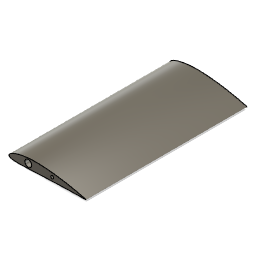
Airfoil v6 (Autodesk Fusion 360 design; units mm, degrees)
Autodesk Fusion 360 part; units mm, degrees
sketch "Esquisse7" plane through (0, 0, 0) normal (0, 0, 1) x (1, 0, 0)
  spline S0 degree 5 poles (0, 0) (-0.0102, 0.0513) (-0.0251, 0.1551) (-0.0316, 0.3133) (-0.0088, 0.5269) (0.0656, 0.7917) (0.1767, 1.0474) (0.3135, 1.2879) (0.4648, 1.5082) (0.6211, 1.7053) (0.7754, 1.8785) (0.9248, 2.03) (1.0699, 2.1643) (1.2127, 2.2866) (1.3565, 2.4023) (1.5042, 2.516) (1.6573, 2.63) (1.8156, 2.7448) (1.9781, 2.8596) (2.143, 2.9726) (2.3089, 3.0823) (2.4745, 3.1876) (2.6395, 3.2884) (2.8042, 3.3853) (2.969, 3.4791) (3.1347, 3.5708) (3.3016, 3.6612) (3.4698, 3.7505) (3.6393, 3.8389) (3.8097, 3.9259) (3.9807, 4.0114) (4.1521, 4.0951) (4.3237, 4.177) (4.4955, 4.2571) (4.6676, 4.3356) (4.8401, 4.4128) (5.0131, 4.4888) (5.1866, 4.5637) (5.3605, 4.6375) (5.535, 4.7103) (5.7098, 4.7821) (5.8849, 4.8527) (6.0602, 4.9221) (6.2358, 4.9905) (6.4117, 5.0579) (6.5879, 5.1242) (6.7643, 5.1896) (6.941, 5.2541) (7.118, 5.3178) (7.2952, 5.3805) (7.4727, 5.4424) (7.6504, 5.5035) (7.8284, 5.5637) (8.0065, 5.6231) (8.1849, 5.6816) (8.3634, 5.7394) (8.5421, 5.7964) (8.7211, 5.8527) (8.9002, 5.9082) (9.0795, 5.963) (9.259, 6.0171) (9.4387, 6.0704) (9.6185, 6.1231) (9.7985, 6.1751) (9.9786, 6.2264) (10.1589, 6.277) (10.3393, 6.3269) (10.5199, 6.3763) (10.7006, 6.4249) (10.8815, 6.473) (11.0625, 6.5204) (11.2436, 6.5672) (11.4249, 6.6134) (11.6063, 6.659) (11.7878, 6.704) (11.9694, 6.7484) (12.1512, 6.7923) (12.333, 6.8355) (12.515, 6.8782) (12.6971, 6.9204) (12.8793, 6.9619) (13.0616, 7.003) (13.2439, 7.0434) (13.4264, 7.0834) (13.609, 7.1228) (13.7917, 7.1617) (13.9745, 7.2) (14.1574, 7.2378) (14.3403, 7.2752) (14.5233, 7.312) (14.7065, 7.3482) (14.8897, 7.384) (15.073, 7.4193) (15.2563, 7.4541) (15.4398, 7.4884) (15.6233, 7.5223) (15.8069, 7.5556) (15.9906, 7.5885) (16.1743, 7.6209) (16.3581, 7.6528) (16.542, 7.6842) (16.726, 7.7152) (16.91, 7.7457) (17.0941, 7.7758) (17.2782, 7.8054) (17.4624, 7.8345) (17.6466, 7.8632) (17.831, 7.8915) (18.0153, 7.9193) (18.1998, 7.9467) (18.3842, 7.9736) (18.5688, 8.0001) (18.7534, 8.0262) (18.938, 8.0519) (19.1227, 8.0771) (19.3074, 8.1019) (19.4922, 8.1262) (19.677, 8.1502) (19.8619, 8.1737) (20.0468, 8.1968) (20.2318, 8.2195) (20.4168, 8.2418) (20.6018, 8.2637) (20.7869, 8.2852) (20.972, 8.3062) (21.1572, 8.3269) (21.3424, 8.3472) (21.5276, 8.3671) (21.7129, 8.3866) (21.8982, 8.4056) (22.0835, 8.4243) (22.2689, 8.4426) (22.4543, 8.4606) (22.6397, 8.4781) (22.8251, 8.4952) (23.0106, 8.512) (23.1961, 8.5284) (23.3817, 8.5444) (23.5673, 8.56) (23.7528, 8.5753) (23.9385, 8.5902) (24.1241, 8.6047) (24.3098, 8.6188) (24.4954, 8.6326) (24.6812, 8.646) (24.8669, 8.659) (25.0526, 8.6717) (25.2384, 8.684) (25.4242, 8.696) (25.61, 8.7076) (25.7958, 8.7188) (25.9816, 8.7297) (26.1675, 8.7402) (26.3534, 8.7504) (26.5392, 8.7602) (26.7251, 8.7696) (26.9111, 8.7788) (27.097, 8.7875) (27.2829, 8.796) (27.4689, 8.804) (27.6548, 8.8118) (27.8408, 8.8191) (28.0268, 8.8262) (28.2127, 8.8329) (28.3987, 8.8393) (28.5847, 8.8453) (28.7707, 8.851) (28.9567, 8.8563) (29.1428, 8.8614) (29.3288, 8.8661) (29.5148, 8.8704) (29.7009, 8.8744) (29.8869, 8.8781) (30.0729, 8.8815) (30.259, 8.8845) (30.445, 8.8873) (30.6311, 8.8896) (30.8171, 8.8917) (31.0032, 8.8934) (31.1892, 8.8949) (31.3753, 8.896) (31.5613, 8.8967) (31.7473, 8.8972) (31.9334, 8.8973) (32.1194, 8.8972) (32.3055, 8.8967) (32.4915, 8.8959) (32.6775, 8.8947) (32.8636, 8.8933) (33.0496, 8.8916) (33.2356, 8.8895) (33.4216, 8.8871) (33.6076, 8.8844) (33.7936, 8.8815) (33.9795, 8.8782) (34.1655, 8.8745) (34.3515, 8.8706) (34.5375, 8.8664) (34.7235, 8.8619) (34.9095, 8.8571) (35.0955, 8.852) (35.2814, 8.8466) (35.4672, 8.8408) (35.6529, 8.8348) (35.8384, 8.8284) (36.0237, 8.8218) (36.2087, 8.8149) (36.3935, 8.8079) (36.5781, 8.8006) (36.7625, 8.7931) (36.9468, 8.7854) (37.131, 8.7775) (37.3152, 8.7695) (37.4995, 8.7612) (37.6838, 8.7528) (37.8681, 8.7442) (38.0525, 8.7353) (38.2369, 8.7263) (38.4212, 8.7171) (38.6055, 8.7078) (38.7898, 8.6982) (38.974, 8.6885) (39.1583, 8.6786) (39.3425, 8.6685) (39.5267, 8.6582) (39.711, 8.6477) (39.8952, 8.6371) (40.0794, 8.6262) (40.2637, 8.6152) (40.4479, 8.604) (40.632, 8.5927) (40.8162, 8.5811) (41.0004, 8.5694) (41.1845, 8.5575) (41.3687, 8.5455) (41.5528, 8.5332) (41.7369, 8.5208) (41.921, 8.5082) (42.1051, 8.4955) (42.2892, 8.4825) (42.4733, 8.4694) (42.6574, 8.4561) (42.8414, 8.4427) (43.0255, 8.4291) (43.2095, 8.4153) (43.3935, 8.4013) (43.5775, 8.3872) (43.7615, 8.3729) (43.9455, 8.3585) (44.1295, 8.3439) (44.3135, 8.3291) (44.4974, 8.3141) (44.6813, 8.299) (44.8653, 8.2837) (45.0492, 8.2683) (45.2331, 8.2527) (45.4169, 8.2369) (45.6008, 8.221) (45.7847, 8.2049) (45.9685, 8.1886) (46.1523, 8.1722) (46.3362, 8.1556) (46.52, 8.1389) (46.7037, 8.122) (46.8875, 8.1049) (47.0713, 8.0877) (47.255, 8.0704) (47.4388, 8.0528) (47.6225, 8.0352) (47.8062, 8.0173) (47.9899, 7.9993) (48.1735, 7.9812) (48.3572, 7.9629) (48.5408, 7.9444) (48.7245, 7.9258) (48.9081, 7.907) (49.0917, 7.8881) (49.2753, 7.869) (49.4589, 7.8498) (49.6424, 7.8304) (49.826, 7.8109) (50.0095, 7.7912) (50.193, 7.7713) (50.3765, 7.7514) (50.56, 7.7312) (50.7434, 7.7109) (50.9269, 7.6905) (51.1103, 7.6699) (51.2937, 7.6492) (51.4771, 7.6283) (51.6605, 7.6073) (51.8439, 7.5861) (52.0272, 7.5648) (52.2106, 7.5433) (52.3939, 7.5217) (52.5772, 7.4999) (52.7605, 7.478) (52.9438, 7.4559) (53.127, 7.4337) (53.3102, 7.4114) (53.4935, 7.3889) (53.6767, 7.3663) (53.8599, 7.3435) (54.043, 7.3206) (54.2262, 7.2975) (54.4093, 7.2743) (54.5924, 7.2509) (54.7755, 7.2274) (54.9586, 7.2038) (55.1417, 7.18) (55.3247, 7.1561) (55.5078, 7.132) (55.6908, 7.1078) (55.8738, 7.0835) (56.0567, 7.059) (56.2397, 7.0344) (56.4226, 7.0096) (56.6056, 6.9847) (56.7885, 6.9597) (56.9714, 6.9345) (57.1542, 6.9091) (57.3371, 6.8837) (57.5199, 6.8581) (57.7027, 6.8323) (57.8855, 6.8065) (58.0683, 6.7805) (58.2511, 6.7543) (58.4338, 6.728) (58.6165, 6.7016) (58.7992, 6.675) (58.9819, 6.6483) (59.1646, 6.6215) (59.3472, 6.5945) (59.5298, 6.5674) (59.7125, 6.5402) (59.895, 6.5128) (60.0776, 6.4853) (60.2602, 6.4576) (60.4427, 6.4298) (60.6252, 6.4019) (60.8077, 6.3739) (60.9902, 6.3457) (61.1726, 6.3174) (61.3551, 6.2889) (61.5375, 6.2603) (61.7199, 6.2316) (61.9022, 6.2027) (62.0846, 6.1737) (62.2669, 6.1446) (62.4492, 6.1153) (62.6315, 6.086) (62.8138, 6.0564) (62.996, 6.0268) (63.1783, 5.997) (63.3605, 5.9671) (63.5427, 5.937) (63.7248, 5.9068) (63.907, 5.8765) (64.0891, 5.846) (64.2712, 5.8155) (64.4533, 5.7848) (64.6354, 5.7539) (64.8174, 5.7229) (64.9995, 5.6918) (65.1815, 5.6606) (65.3634, 5.6292) (65.5454, 5.5977) (65.7273, 5.5661) (65.9092, 5.5343) (66.0911, 5.5024) (66.273, 5.4704) (66.4549, 5.4382) (66.6367, 5.406) (66.8185, 5.3736) (67.0003, 5.341) (67.1821, 5.3083) (67.3638, 5.2755) (67.5455, 5.2426) (67.7272, 5.2095) (67.9089, 5.1763) (68.0906, 5.143) (68.2722, 5.1096) (68.4538, 5.076) (68.6354, 5.0423) (68.8169, 5.0084) (68.9985, 4.9744) (69.18, 4.9403) (69.3615, 4.9061) (69.543, 4.8718) (69.7244, 4.8373) (69.9059, 4.8027) (70.0873, 4.7679) (70.2686, 4.733) (70.45, 4.698) (70.6313, 4.6629) (70.8127, 4.6276) (70.9939, 4.5922) (71.1752, 4.5567) (71.3564, 4.5211) (71.5377, 4.4853) (71.7189, 4.4494) (71.9, 4.4133) (72.0812, 4.3772) (72.2623, 4.3409) (72.4434, 4.3045) (72.6245, 4.2679) (72.8055, 4.2312) (72.9865, 4.1944) (73.1675, 4.1575) (73.3485, 4.1204) (73.5295, 4.0832) (73.7104, 4.0459) (73.8913, 4.0084) (74.0722, 3.9708) (74.253, 3.9331) (74.4339, 3.8953) (74.6147, 3.8573) (74.7954, 3.8192) (74.9762, 3.781) (75.1569, 3.7426) (75.3376, 3.7041) (75.5183, 3.6655) (75.6989, 3.6268) (75.8796, 3.5879) (76.0602, 3.5489) (76.2407, 3.5098) (76.4213, 3.4705) (76.6018, 3.4311) (76.7823, 3.3916) (76.9628, 3.3519) (77.1432, 3.3122) (77.3236, 3.2722) (77.504, 3.2322) (77.6844, 3.192) (77.8647, 3.1517) (78.045, 3.1113) (78.2253, 3.0707) (78.4056, 3.03) (78.5858, 2.9892) (78.766, 2.9483) (78.9462, 2.9072) (79.1264, 2.866) (79.3065, 2.8246) (79.4866, 2.7831) (79.6666, 2.7415) (79.8467, 2.6998) (80.0267, 2.6579) (80.2067, 2.6159) (80.3866, 2.5738) (80.5666, 2.5316) (80.7465, 2.4892) (80.9263, 2.4466) (81.1062, 2.404) (81.2859, 2.3612) (81.4657, 2.3182) (81.6455, 2.2752) (81.8252, 2.232) (82.0049, 2.1887) (82.1847, 2.1453) (82.3643, 2.1017) (82.544, 2.058) (82.7235, 2.0142) (82.903, 1.9701) (83.0824, 1.926) (83.2618, 1.8817) (83.4412, 1.8373) (83.6208, 1.7928) (83.8003, 1.7483) (83.98, 1.7036) (84.1595, 1.6588) (84.3389, 1.6138) (84.518, 1.5685) (84.6968, 1.5229) (84.8754, 1.4772) (85.0541, 1.4313) (85.2332, 1.3855) (85.4128, 1.3399) (85.5929, 1.2945) (85.7733, 1.2492) (85.9534, 1.2035) (86.1326, 1.1573) (86.3106, 1.1101) (86.4872, 1.0621) (86.663, 1.0135) (86.8393, 0.9651) (87.0176, 0.9177) (87.1988, 0.8719) (87.3831, 0.8277) (87.569, 0.7843) (87.7535, 0.7401) (87.9336, 0.6931) (88.1067, 0.642) (88.2727, 0.5866) (88.4345, 0.5288) (88.5991, 0.4726) (88.7741, 0.4223) (88.9652, 0.3811) (89.1737, 0.3493) (89.3935, 0.3227) (89.61, 0.292) (89.8042, 0.2472) (89.9561, 0.181) (90.0488, 0.0924) (90.0719, -0.0084) (90.0246, -0.1002) (89.9133, -0.1623) (89.7503, -0.1873) (89.5518, -0.1807) (89.3352, -0.1543) (89.1161, -0.123) (88.9064, -0.0997) (88.7111, -0.0903) (88.529, -0.094) (88.3554, -0.1064) (88.1842, -0.1213) (88.0098, -0.133) (87.8296, -0.139) (87.6438, -0.1392) (87.4543, -0.1358) (87.2637, -0.1313) (87.0746, -0.1282) (86.8879, -0.1277) (86.7036, -0.1296) (86.521, -0.1331) (86.3389, -0.1371) (86.1561, -0.1406) (85.9723, -0.143) (85.7875, -0.1444) (85.602, -0.1451) (85.4164, -0.1457) (85.231, -0.1465) (85.0461, -0.1478) (84.8616, -0.1496) (84.6775, -0.1518) (84.4934, -0.154) (84.3093, -0.1562) (84.1249, -0.1581) (83.9404, -0.16) (83.7558, -0.1617) (83.5711, -0.1634) (83.3866, -0.1652) (83.2021, -0.1671) (83.0177, -0.1691) (82.8334, -0.1712) (82.6491, -0.1734) (82.4648, -0.1755) (82.2805, -0.1777) (82.0961, -0.1798) (81.9118, -0.1819) (81.7274, -0.1841) (81.5431, -0.1863) (81.3588, -0.1886) (81.1745, -0.1909) (80.9903, -0.1932) (80.8061, -0.1956) (80.6219, -0.198) (80.4377, -0.2004) (80.2535, -0.2029) (80.0693, -0.2054) (79.8851, -0.2079) (79.7009, -0.2104) (79.5168, -0.213) (79.3326, -0.2156) (79.1485, -0.2183) (78.9644, -0.221) (78.7803, -0.2237) (78.5962, -0.2264) (78.4122, -0.2292) (78.2281, -0.232) (78.0441, -0.2348) (77.86, -0.2377) (77.676, -0.2406) (77.492, -0.2436) (77.308, -0.2465) (77.124, -0.2495) (76.9401, -0.2526) (76.7561, -0.2556) (76.5722, -0.2588) (76.3882, -0.2619) (76.2043, -0.2651) (76.0204, -0.2683) (75.8365, -0.2715) (75.6526, -0.2748) (75.4688, -0.2781) (75.2849, -0.2814) (75.1011, -0.2848) (74.9173, -0.2882) (74.7334, -0.2917) (74.5496, -0.2951) (74.3658, -0.2987) (74.1821, -0.3022) (73.9983, -0.3058) (73.8145, -0.3094) (73.6308, -0.3131) (73.4471, -0.3167) (73.2633, -0.3205) (73.0796, -0.3242) (72.8959, -0.328) (72.7123, -0.3318) (72.5286, -0.3357) (72.3449, -0.3396) (72.1613, -0.3435) (71.9776, -0.3475) (71.794, -0.3515) (71.6104, -0.3555) (71.4268, -0.3596) (71.2432, -0.3637) (71.0596, -0.3678) (70.8761, -0.372) (70.6925, -0.3762) (70.509, -0.3804) (70.3254, -0.3847) (70.1419, -0.389) (69.9584, -0.3933) (69.7749, -0.3977) (69.5914, -0.4021) (69.408, -0.4066) (69.2245, -0.4111) (69.041, -0.4156) (68.8576, -0.4201) (68.6742, -0.4247) (68.4908, -0.4293) (68.3074, -0.434) (68.124, -0.4387) (67.9406, -0.4434) (67.7572, -0.4481) (67.5739, -0.4529) (67.3905, -0.4578) (67.2072, -0.4626) (67.0238, -0.4675) (66.8405, -0.4724) (66.6572, -0.4774) (66.4739, -0.4824) (66.2906, -0.4874) (66.1074, -0.4925) (65.9241, -0.4976) (65.7409, -0.5027) (65.5576, -0.5079) (65.3744, -0.5131) (65.1912, -0.5183) (65.008, -0.5236) (64.8248, -0.5289) (64.6416, -0.5342) (64.4584, -0.5396) (64.2753, -0.545) (64.0921, -0.5504) (63.909, -0.5558) (63.7258, -0.5613) (63.5427, -0.5669) (63.3596, -0.5724) (63.1765, -0.578) (62.9934, -0.5836) (62.8103, -0.5893) (62.6273, -0.595) (62.4442, -0.6007) (62.2612, -0.6064) (62.0781, -0.6122) (61.8951, -0.618) (61.7121, -0.6239) (61.5291, -0.6297) (61.3461, -0.6356) (61.1631, -0.6416) (60.9801, -0.6475) (60.7971, -0.6535) (60.6142, -0.6596) (60.4312, -0.6656) (60.2483, -0.6717) (60.0654, -0.6778) (59.8825, -0.6839) (59.6996, -0.6901) (59.5167, -0.6963) (59.3338, -0.7025) (59.1509, -0.7088) (58.968, -0.7151) (58.7852, -0.7214) (58.6023, -0.7277) (58.4195, -0.7341) (58.2367, -0.7405) (58.0539, -0.7469) (57.8711, -0.7534) (57.6883, -0.7599) (57.5055, -0.7664) (57.3227, -0.7729) (57.1399, -0.7795) (56.9572, -0.786) (56.7744, -0.7927) (56.5917, -0.7993) (56.4089, -0.8059) (56.2262, -0.8126) (56.0435, -0.8193) (55.8608, -0.8261) (55.6781, -0.8328) (55.4954, -0.8396) (55.3127, -0.8464) (55.1301, -0.8532) (54.9474, -0.8601) (54.7648, -0.867) (54.5821, -0.8739) (54.3995, -0.8808) (54.2169, -0.8877) (54.0343, -0.8947) (53.8517, -0.9017) (53.6691, -0.9087) (53.4865, -0.9157) (53.3039, -0.9228) (53.1213, -0.9298) (52.9388, -0.9369) (52.7562, -0.944) (52.5737, -0.9511) (52.3911, -0.9583) (52.2086, -0.9654) (52.0261, -0.9726) (51.8436, -0.9798) (51.6611, -0.987) (51.4786, -0.9943) (51.2961, -1.0015) (51.1136, -1.0088) (50.9311, -1.0161) (50.7487, -1.0233) (50.5662, -1.0307) (50.3838, -1.038) (50.2013, -1.0453) (50.0189, -1.0527) (49.8365, -1.0601) (49.6541, -1.0674) (49.4717, -1.0748) (49.2893, -1.0822) (49.1069, -1.0897) (48.9245, -1.0971) (48.7421, -1.1045) (48.5598, -1.112) (48.3774, -1.1194) (48.1951, -1.1269) (48.0127, -1.1344) (47.8304, -1.1419) (47.648, -1.1494) (47.4657, -1.1569) (47.2834, -1.1644) (47.1011, -1.1719) (46.9188, -1.1795) (46.7365, -1.187) (46.5542, -1.1946) (46.3719, -1.2021) (46.1896, -1.2097) (46.0074, -1.2172) (45.8251, -1.2248) (45.6429, -1.2323) (45.4606, -1.2399) (45.2784, -1.2475) (45.0961, -1.2551) (44.9139, -1.2626) (44.7317, -1.2702) (44.5495, -1.2778) (44.3673, -1.2853) (44.1851, -1.2929) (44.0029, -1.3005) (43.8207, -1.3081) (43.6385, -1.3156) (43.4563, -1.3232) (43.2741, -1.3308) (43.092, -1.3383) (42.9098, -1.3459) (42.7276, -1.3534) (42.5455, -1.361) (42.3633, -1.3685) (42.1812, -1.376) (41.9991, -1.3835) (41.8169, -1.3911) (41.6348, -1.3986) (41.4527, -1.4061) (41.2706, -1.4135) (41.0885, -1.421) (40.9064, -1.4285) (40.7243, -1.4359) (40.5422, -1.4434) (40.3601, -1.4508) (40.178, -1.4582) (39.9959, -1.4656) (39.8138, -1.473) (39.6318, -1.4803) (39.4497, -1.4877) (39.2676, -1.495) (39.0856, -1.5023) (38.9035, -1.5096) (38.7214, -1.5169) (38.5394, -1.5241) (38.3573, -1.5314) (38.1753, -1.5386) (37.9933, -1.5457) (37.8114, -1.5529) (37.6294, -1.56) (37.4473, -1.5672) (37.2652, -1.5742) (37.083, -1.5813) (36.9009, -1.5883) (36.7188, -1.5953) (36.5368, -1.6023) (36.3551, -1.6093) (36.1735, -1.6162) (35.9922, -1.6231) (35.8112, -1.6301) (35.6304, -1.6371) (35.4497, -1.6441) (35.2692, -1.6513) (35.0887, -1.6585) (34.9083, -1.6658) (34.7279, -1.6732) (34.5475, -1.6806) (34.3671, -1.6881) (34.1867, -1.6956) (34.0063, -1.7032) (33.8259, -1.7109) (33.6455, -1.7186) (33.4651, -1.7264) (33.2847, -1.7342) (33.1043, -1.7421) (32.9239, -1.75) (32.7436, -1.758) (32.5632, -1.7661) (32.3829, -1.7742) (32.2025, -1.7823) (32.0221, -1.7905) (31.8418, -1.7988) (31.6614, -1.807) (31.4811, -1.8154) (31.3007, -1.8238) (31.1204, -1.8322) (30.9401, -1.8406) (30.7597, -1.8491) (30.5794, -1.8577) (30.3991, -1.8663) (30.2187, -1.8749) (30.0384, -1.8835) (29.8581, -1.8922) (29.6777, -1.9009) (29.4974, -1.9097) (29.3171, -1.9185) (29.1368, -1.9273) (28.9564, -1.9361) (28.7761, -1.945) (28.5958, -1.9538) (28.4154, -1.9628) (28.2351, -1.9717) (28.0547, -1.9806) (27.8744, -1.9896) (27.694, -1.9986) (27.5137, -2.0076) (27.3333, -2.0166) (27.153, -2.0257) (26.9726, -2.0347) (26.7922, -2.0438) (26.6119, -2.0528) (26.4315, -2.0619) (26.2511, -2.071) (26.0707, -2.0801) (25.8903, -2.0891) (25.7099, -2.0982) (25.5295, -2.1073) (25.3491, -2.1164) (25.1686, -2.1255) (24.9882, -2.1345) (24.8077, -2.1436) (24.6273, -2.1527) (24.4468, -2.1617) (24.2663, -2.1707) (24.0858, -2.1797) (23.9053, -2.1887) (23.7248, -2.1977) (23.5443, -2.2067) (23.3637, -2.2156) (23.1832, -2.2245) (23.0026, -2.2334) (22.822, -2.2422) (22.6414, -2.251) (22.4608, -2.2598) (22.2802, -2.2686) (22.0995, -2.2773) (21.9189, -2.2859) (21.7382, -2.2945) (21.5575, -2.3031) (21.3768, -2.3117) (21.1961, -2.3201) (21.0153, -2.3286) (20.8345, -2.3369) (20.6537, -2.3452) (20.4729, -2.3535) (20.2921, -2.3617) (20.1112, -2.3698) (19.9304, -2.3779) (19.7495, -2.3858) (19.5685, -2.3937) (19.3876, -2.4016) (19.2066, -2.4093) (19.0256, -2.417) (18.8446, -2.4246) (18.6635, -2.4321) (18.4824, -2.4395) (18.3013, -2.4468) (18.1202, -2.454) (17.939, -2.4611) (17.7578, -2.4681) (17.5766, -2.4749) (17.3953, -2.4817) (17.2141, -2.4883) (17.0327, -2.4949) (16.8514, -2.5013) (16.67, -2.5075) (16.4885, -2.5137) (16.3071, -2.5197) (16.1256, -2.5255) (15.944, -2.5312) (15.7625, -2.5368) (15.5808, -2.5422) (15.3992, -2.5474) (15.2175, -2.5525) (15.0358, -2.5574) (14.854, -2.5621) (14.6722, -2.5667) (14.4903, -2.571) (14.3084, -2.5752) (14.1264, -2.5792) (13.9444, -2.5829) (13.7623, -2.5865) (13.5802, -2.5898) (13.3981, -2.5929) (13.2159, -2.5958) (13.0336, -2.5984) (12.8513, -2.6008) (12.669, -2.6029) (12.4865, -2.6048) (12.3041, -2.6064) (12.1215, -2.6077) (11.939, -2.6088) (11.7563, -2.6095) (11.5736, -2.61) (11.3908, -2.6101) (11.208, -2.6099) (11.0251, -2.6094) (10.8421, -2.6085) (10.6591, -2.6072) (10.476, -2.6056) (10.2928, -2.6036) (10.1096, -2.6013) (9.9263, -2.5985) (9.7429, -2.5953) (9.5595, -2.5916) (9.376, -2.5875) (9.1923, -2.583) (9.0086, -2.5779) (8.8249, -2.5724) (8.641, -2.5663) (8.457, -2.5597) (8.273, -2.5525) (8.0889, -2.5447) (7.9047, -2.5364) (7.7205, -2.5274) (7.5362, -2.5178) (7.3517, -2.5075) (7.1671, -2.4965) (6.9824, -2.4846) (6.7975, -2.472) (6.6124, -2.4585) (6.4274, -2.4443) (6.2424, -2.4292) (6.0574, -2.4133) (5.8725, -2.3965) (5.6875, -2.3786) (5.5022, -2.3596) (5.3165, -2.3392) (5.1302, -2.3175) (4.9435, -2.2942) (4.7566, -2.2696) (4.5701, -2.2438) (4.3842, -2.2169) (4.1991, -2.1888) (4.0147, -2.1594) (3.8303, -2.1283) (3.645, -2.0947) (3.458, -2.0579) (3.2686, -2.0177) (3.0772, -1.9738) (2.8851, -1.9267) (2.6943, -1.8774) (2.5072, -1.8266) (2.3251, -1.7749) (2.1481, -1.7218) (1.974, -1.6658) (1.7983, -1.6038) (1.616, -1.5321) (1.4229, -1.4466) (1.217, -1.3435) (0.9996, -1.2194) (0.7775, -1.0725) (0.5607, -0.9016) (0.3614, -0.7072) (0.1922, -0.4906) (0.09, -0.3017) (0.0358, -0.153) (0.0102, -0.0513) (0, 0) knots 0 0 0 0 0 0 0.00100503 0.00201005 0.00301508 0.0040201 0.00502513 0.00603015 0.00703518 0.0080402 0.00904523 0.01005025 0.01105528 0.0120603 0.01306533 0.01407035 0.01507538 0.0160804 0.01708543 0.01809045 0.01909548 0.0201005 0.02110553 0.02211055 0.02311558 0.0241206 0.02512563 0.02613065 0.02713568 0.0281407 0.02914573 0.03015075 0.03115578 0.0321608 0.03316583 0.03417085 0.03517588 0.0361809 0.03718593 0.03819095 0.03919598 0.04020101 0.04120603 0.04221106 0.04321608 0.04422111 0.04522613 0.04623116 0.04723618 0.04824121 0.04924623 0.05025126 0.05125628 0.05226131 0.05326633 0.05427136 0.05527638 0.05628141 0.05728643 0.05829146 0.05929648 0.06030151 0.06130653 0.06231156 0.06331658 0.06432161 0.06532663 0.06633166 0.06733668 0.06834171 0.06934673 0.07035176 0.07135678 0.07236181 0.07336683 0.07437186 0.07537688 0.07638191 0.07738693 0.07839196 0.07939698 0.08040201 0.08140704 0.08241206 0.08341709 0.08442211 0.08542714 0.08643216 0.08743719 0.08844221 0.08944724 0.09045226 0.09145729 0.09246231 0.09346734 0.09447236 0.09547739 0.09648241 0.09748744 0.09849246 0.09949749 0.10050251 0.10150754 0.10251256 0.10351759 0.10452261 0.10552764 0.10653266 0.10753769 0.10854271 0.10954774 0.11055276 0.11155779 0.11256281 0.11356784 0.11457286 0.11557789 0.11658291 0.11758794 0.11859296 0.11959799 0.12060302 0.12160804 0.12261307 0.12361809 0.12462312 0.12562814 0.12663317 0.12763819 0.12864322 0.12964824 0.13065327 0.13165829 0.13266332 0.13366834 0.13467337 0.13567839 0.13668342 0.13768844 0.13869347 0.13969849 0.14070352 0.14170854 0.14271357 0.14371859 0.14472362 0.14572864 0.14673367 0.14773869 0.14874372 0.14974874 0.15075377 0.15175879 0.15276382 0.15376884 0.15477387 0.15577889 0.15678392 0.15778894 0.15879397 0.15979899 0.16080402 0.16180905 0.16281407 0.1638191 0.16482412 0.16582915 0.16683417 0.1678392 0.16884422 0.16984925 0.17085427 0.1718593 0.17286432 0.17386935 0.17487437 0.1758794 0.17688442 0.17788945 0.17889447 0.1798995 0.18090452 0.18190955 0.18291457 0.1839196 0.18492462 0.18592965 0.18693467 0.1879397 0.18894472 0.18994975 0.19095477 0.1919598 0.19296482 0.19396985 0.19497487 0.1959799 0.19698492 0.19798995 0.19899497 0.2 0.20100503 0.20201005 0.20301508 0.2040201 0.20502513 0.20603015 0.20703518 0.2080402 0.20904523 0.21005025 0.21105528 0.2120603 0.21306533 0.21407035 0.21507538 0.2160804 0.21708543 0.21809045 0.21909548 0.2201005 0.22110553 0.22211055 0.22311558 0.2241206 0.22512563 0.22613065 0.22713568 0.2281407 0.22914573 0.23015075 0.23115578 0.2321608 0.23316583 0.23417085 0.23517588 0.2361809 0.23718593 0.23819095 0.23919598 0.24020101 0.24120603 0.24221106 0.24321608 0.24422111 0.24522613 0.24623116 0.24723618 0.24824121 0.24924623 0.25025126 0.25125628 0.25226131 0.25326633 0.25427136 0.25527638 0.25628141 0.25728643 0.25829146 0.25929648 0.26030151 0.26130653 0.26231156 0.26331658 0.26432161 0.26532663 0.26633166 0.26733668 0.26834171 0.26934673 0.27035176 0.27135678 0.27236181 0.27336683 0.27437186 0.27537688 0.27638191 0.27738693 0.27839196 0.27939698 0.28040201 0.28140704 0.28241206 0.28341709 0.28442211 0.28542714 0.28643216 0.28743719 0.28844221 0.28944724 0.29045226 0.29145729 0.29246231 0.29346734 0.29447236 0.29547739 0.29648241 0.29748744 0.29849246 0.29949749 0.30050251 0.30150754 0.30251256 0.30351759 0.30452261 0.30552764 0.30653266 0.30753769 0.30854271 0.30954774 0.31055276 0.31155779 0.31256281 0.31356784 0.31457286 0.31557789 0.31658291 0.31758794 0.31859296 0.31959799 0.32060302 0.32160804 0.32261307 0.32361809 0.32462312 0.32562814 0.32663317 0.32763819 0.32864322 0.32964824 0.33065327 0.33165829 0.33266332 0.33366834 0.33467337 0.33567839 0.33668342 0.33768844 0.33869347 0.33969849 0.34070352 0.34170854 0.34271357 0.34371859 0.34472362 0.34572864 0.34673367 0.34773869 0.34874372 0.34974874 0.35075377 0.35175879 0.35276382 0.35376884 0.35477387 0.35577889 0.35678392 0.35778894 0.35879397 0.35979899 0.36080402 0.36180905 0.36281407 0.3638191 0.36482412 0.36582915 0.36683417 0.3678392 0.36884422 0.36984925 0.37085427 0.3718593 0.37286432 0.37386935 0.37487437 0.3758794 0.37688442 0.37788945 0.37889447 0.3798995 0.38090452 0.38190955 0.38291457 0.3839196 0.38492462 0.38592965 0.38693467 0.3879397 0.38894472 0.38994975 0.39095477 0.3919598 0.39296482 0.39396985 0.39497487 0.3959799 0.39698492 0.39798995 0.39899497 0.4 0.40100503 0.40201005 0.40301508 0.4040201 0.40502513 0.40603015 0.40703518 0.4080402 0.40904523 0.41005025 0.41105528 0.4120603 0.41306533 0.41407035 0.41507538 0.4160804 0.41708543 0.41809045 0.41909548 0.4201005 0.42110553 0.42211055 0.42311558 0.4241206 0.42512563 0.42613065 0.42713568 0.4281407 0.42914573 0.43015075 0.43115578 0.4321608 0.43316583 0.43417085 0.43517588 0.4361809 0.43718593 0.43819095 0.43919598 0.44020101 0.44120603 0.44221106 0.44321608 0.44422111 0.44522613 0.44623116 0.44723618 0.44824121 0.44924623 0.45025126 0.45125628 0.45226131 0.45326633 0.45427136 0.45527638 0.45628141 0.45728643 0.45829146 0.45929648 0.46030151 0.46130653 0.46231156 0.46331658 0.46432161 0.46532663 0.46633166 0.46733668 0.46834171 0.46934673 0.47035176 0.47135678 0.47236181 0.47336683 0.47437186 0.47537688 0.47638191 0.47738693 0.47839196 0.47939698 0.48040201 0.48140704 0.48241206 0.48341709 0.48442211 0.48542714 0.48643216 0.48743719 0.48844221 0.48944724 0.49045226 0.49145729 0.49246231 0.49346734 0.49447236 0.49547739 0.49648241 0.49748744 0.49849246 0.49949749 0.50050251 0.50150754 0.50251256 0.50351759 0.50452261 0.50552764 0.50653266 0.50753769 0.50854271 0.50954774 0.51055276 0.51155779 0.51256281 0.51356784 0.51457286 0.51557789 0.51658291 0.51758794 0.51859296 0.51959799 0.52060302 0.52160804 0.52261307 0.52361809 0.52462312 0.52562814 0.52663317 0.52763819 0.52864322 0.52964824 0.53065327 0.53165829 0.53266332 0.53366834 0.53467337 0.53567839 0.53668342 0.53768844 0.53869347 0.53969849 0.54070352 0.54170854 0.54271357 0.54371859 0.54472362 0.54572864 0.54673367 0.54773869 0.54874372 0.54974874 0.55075377 0.55175879 0.55276382 0.55376884 0.55477387 0.55577889 0.55678392 0.55778894 0.55879397 0.55979899 0.56080402 0.56180905 0.56281407 0.5638191 0.56482412 0.56582915 0.56683417 0.5678392 0.56884422 0.56984925 0.57085427 0.5718593 0.57286432 0.57386935 0.57487437 0.5758794 0.57688442 0.57788945 0.57889447 0.5798995 0.58090452 0.58190955 0.58291457 0.5839196 0.58492462 0.58592965 0.58693467 0.5879397 0.58894472 0.58994975 0.59095477 0.5919598 0.59296482 0.59396985 0.59497487 0.5959799 0.59698492 0.59798995 0.59899497 0.6 0.60100503 0.60201005 0.60301508 0.6040201 0.60502513 0.60603015 0.60703518 0.6080402 0.60904523 0.61005025 0.61105528 0.6120603 0.61306533 0.61407035 0.61507538 0.6160804 0.61708543 0.61809045 0.61909548 0.6201005 0.62110553 0.62211055 0.62311558 0.6241206 0.62512563 0.62613065 0.62713568 0.6281407 0.62914573 0.63015075 0.63115578 0.6321608 0.63316583 0.63417085 0.63517588 0.6361809 0.63718593 0.63819095 0.63919598 0.64020101 0.64120603 0.64221106 0.64321608 0.64422111 0.64522613 0.64623116 0.64723618 0.64824121 0.64924623 0.65025126 0.65125628 0.65226131 0.65326633 0.65427136 0.65527638 0.65628141 0.65728643 0.65829146 0.65929648 0.66030151 0.66130653 0.66231156 0.66331658 0.66432161 0.66532663 0.66633166 0.66733668 0.66834171 0.66934673 0.67035176 0.67135678 0.67236181 0.67336683 0.67437186 0.67537688 0.67638191 0.67738693 0.67839196 0.67939698 0.68040201 0.68140704 0.68241206 0.68341709 0.68442211 0.68542714 0.68643216 0.68743719 0.68844221 0.68944724 0.69045226 0.69145729 0.69246231 0.69346734 0.69447236 0.69547739 0.69648241 0.69748744 0.69849246 0.69949749 0.70050251 0.70150754 0.70251256 0.70351759 0.70452261 0.70552764 0.70653266 0.70753769 0.70854271 0.70954774 0.71055276 0.71155779 0.71256281 0.71356784 0.71457286 0.71557789 0.71658291 0.71758794 0.71859296 0.71959799 0.72060302 0.72160804 0.72261307 0.72361809 0.72462312 0.72562814 0.72663317 0.72763819 0.72864322 0.72964824 0.73065327 0.73165829 0.73266332 0.73366834 0.73467337 0.73567839 0.73668342 0.73768844 0.73869347 0.73969849 0.74070352 0.74170854 0.74271357 0.74371859 0.74472362 0.74572864 0.74673367 0.74773869 0.74874372 0.74974874 0.75075377 0.75175879 0.75276382 0.75376884 0.75477387 0.75577889 0.75678392 0.75778894 0.75879397 0.75979899 0.76080402 0.76180905 0.76281407 0.7638191 0.76482412 0.76582915 0.76683417 0.7678392 0.76884422 0.76984925 0.77085427 0.7718593 0.77286432 0.77386935 0.77487437 0.7758794 0.77688442 0.77788945 0.77889447 0.7798995 0.78090452 0.78190955 0.78291457 0.7839196 0.78492462 0.78592965 0.78693467 0.7879397 0.78894472 0.78994975 0.79095477 0.7919598 0.79296482 0.79396985 0.79497487 0.7959799 0.79698492 0.79798995 0.79899497 0.8 0.80100503 0.80201005 0.80301508 0.8040201 0.80502513 0.80603015 0.80703518 0.8080402 0.80904523 0.81005025 0.81105528 0.8120603 0.81306533 0.81407035 0.81507538 0.8160804 0.81708543 0.81809045 0.81909548 0.8201005 0.82110553 0.82211055 0.82311558 0.8241206 0.82512563 0.82613065 0.82713568 0.8281407 0.82914573 0.83015075 0.83115578 0.8321608 0.83316583 0.83417085 0.83517588 0.8361809 0.83718593 0.83819095 0.83919598 0.84020101 0.84120603 0.84221106 0.84321608 0.84422111 0.84522613 0.84623116 0.84723618 0.84824121 0.84924623 0.85025126 0.85125628 0.85226131 0.85326633 0.85427136 0.85527638 0.85628141 0.85728643 0.85829146 0.85929648 0.86030151 0.86130653 0.86231156 0.86331658 0.86432161 0.86532663 0.86633166 0.86733668 0.86834171 0.86934673 0.87035176 0.87135678 0.87236181 0.87336683 0.87437186 0.87537688 0.87638191 0.87738693 0.87839196 0.87939698 0.88040201 0.88140704 0.88241206 0.88341709 0.88442211 0.88542714 0.88643216 0.88743719 0.88844221 0.88944724 0.89045226 0.89145729 0.89246231 0.89346734 0.89447236 0.89547739 0.89648241 0.89748744 0.89849246 0.89949749 0.90050251 0.90150754 0.90251256 0.90351759 0.90452261 0.90552764 0.90653266 0.90753769 0.90854271 0.90954774 0.91055276 0.91155779 0.91256281 0.91356784 0.91457286 0.91557789 0.91658291 0.91758794 0.91859296 0.91959799 0.92060302 0.92160804 0.92261307 0.92361809 0.92462312 0.92562814 0.92663317 0.92763819 0.92864322 0.92964824 0.93065327 0.93165829 0.93266332 0.93366834 0.93467337 0.93567839 0.93668342 0.93768844 0.93869347 0.93969849 0.94070352 0.94170854 0.94271357 0.94371859 0.94472362 0.94572864 0.94673367 0.94773869 0.94874372 0.94974874 0.95075377 0.95175879 0.95276382 0.95376884 0.95477387 0.95577889 0.95678392 0.95778894 0.95879397 0.95979899 0.96080402 0.96180905 0.96281407 0.9638191 0.96482412 0.96582915 0.96683417 0.9678392 0.96884422 0.96984925 0.97085427 0.9718593 0.97286432 0.97386935 0.97487437 0.9758794 0.97688442 0.97788945 0.97889447 0.9798995 0.98090452 0.98190955 0.98291457 0.9839196 0.98492462 0.98592965 0.98693467 0.9879397 0.98894472 0.98994975 0.99095477 0.9919598 0.99296482 0.99396985 0.99497487 0.9959799 0.99698492 0.99798995 0.99899497 1 1 1 1 1 1
  circle A0 centre (22.5, 3.09) radius 4
  line L0 (-9, 0) -> (97, 0) construction
  line L1 (0, 19.781) -> (0, -12.219) construction
  circle A1 centre (50.5, 3.09) radius 1.625
  line L2 (22.5, 3.09) -> (50.5, 3.09) construction
  point P0 (0.6143, 1.6917)
  point P1 (1.4201, 2.4507)
  point P2 (2.2605, 3.0497)
  point P3 (3.12, 3.5623)
  point P4 (3.9924, 4.0167)
  point P5 (4.8743, 4.4276)
  point P6 (5.7638, 4.8037)
  point P7 (6.6594, 5.1506)
  point P8 (7.5602, 5.4724)
  point P9 (8.4655, 5.7719)
  point P10 (9.3747, 6.0513)
  point P11 (10.2872, 6.3124)
  point P12 (11.2028, 6.5566)
  point P13 (12.121, 6.7849)
  point P14 (13.0415, 6.9983)
  point P15 (13.9642, 7.1977)
  point P16 (14.8888, 7.3837)
  point P17 (15.8151, 7.557)
  point P18 (16.7429, 7.7179)
  point P19 (17.6721, 7.8671)
  point P20 (18.6025, 8.0048)
  point P21 (19.534, 8.1316)
  point P22 (20.4664, 8.2476)
  point P23 (21.3997, 8.3533)
  point P24 (22.3336, 8.4489)
  point P25 (23.2683, 8.5346)
  point P26 (24.2034, 8.6107)
  point P27 (25.139, 8.6774)
  point P28 (26.0749, 8.7349)
  point P29 (27.0112, 8.7834)
  point P30 (27.9476, 8.8231)
  point P31 (28.8841, 8.8542)
  point P32 (29.8208, 8.8768)
  point P33 (30.7574, 8.891)
  point P34 (31.694, 8.897)
  point P35 (32.6305, 8.895)
  point P36 (33.5668, 8.885)
  point P37 (34.5028, 8.8672)
  point P38 (35.4387, 8.8417)
  point P39 (36.3683, 8.8088)
  point P40 (37.289, 8.7706)
  point P41 (38.2095, 8.7276)
  point P42 (39.1298, 8.6801)
  point P43 (40.0499, 8.6279)
  point P44 (40.9697, 8.5713)
  point P45 (41.8893, 8.5104)
  point P46 (42.8087, 8.4451)
  point P47 (43.7278, 8.3755)
  point P48 (44.6466, 8.3018)
  point P49 (45.5651, 8.224)
  point P50 (46.4833, 8.1422)
  point P51 (47.4011, 8.0564)
  point P52 (48.3187, 7.9667)
  point P53 (49.2359, 7.8731)
  point P54 (50.1527, 7.7757)
  point P55 (51.0692, 7.6745)
  point P56 (51.9853, 7.5696)
  point P57 (52.901, 7.4611)
  point P58 (53.8163, 7.3489)
  point P59 (54.7313, 7.2331)
  point P60 (55.6458, 7.1138)
  point P61 (56.5599, 6.9909)
  point P62 (57.4735, 6.8646)
  point P63 (58.3868, 6.7348)
  point P64 (59.2996, 6.6015)
  point P65 (60.2119, 6.4649)
  point P66 (61.1238, 6.3249)
  point P67 (62.0352, 6.1816)
  point P68 (62.9462, 6.0349)
  point P69 (63.8566, 5.8849)
  point P70 (64.7666, 5.7316)
  point P71 (65.6761, 5.575)
  point P72 (66.5851, 5.4151)
  point P73 (67.4935, 5.252)
  point P74 (68.4015, 5.0856)
  point P75 (69.3089, 4.916)
  point P76 (70.2158, 4.7432)
  point P77 (71.1221, 4.5671)
  point P78 (72.0279, 4.3878)
  point P79 (72.9332, 4.2052)
  point P80 (73.8379, 4.0195)
  point P81 (74.742, 3.8305)
  point P82 (75.6455, 3.6382)
  point P83 (76.5484, 3.4427)
  point P84 (77.4508, 3.244)
  point P85 (78.3525, 3.042)
  point P86 (79.2536, 2.8367)
  point P87 (80.1541, 2.6282)
  point P88 (81.0539, 2.4163)
  point P89 (81.9531, 2.2012)
  point P90 (82.8517, 1.9827)
  point P91 (83.7496, 1.7609)
  point P92 (84.6468, 1.5357)
  point P93 (85.5433, 1.3071)
  point P94 (86.4391, 1.0751)
  point P95 (87.3341, 0.8396)
  point P96 (88.2285, 0.6007)
  point P97 (89.1221, 0.3583)
  point P98 (90.015, 0.1124)
  point P99 (89.985, -0.1124)
  point P100 (89.0597, -0.1179)
  point P101 (88.1351, -0.124)
  point P102 (87.2113, -0.1307)
  point P103 (86.2882, -0.138)
  point P104 (85.3658, -0.146)
  point P105 (84.4442, -0.1546)
  point P106 (83.5232, -0.1639)
  point P107 (82.6029, -0.1739)
  point P108 (81.6832, -0.1847)
  point P109 (80.7642, -0.1962)
  point P110 (79.8459, -0.2084)
  point P111 (78.9282, -0.2215)
  point P112 (78.0111, -0.2354)
  point P113 (77.0947, -0.25)
  point P114 (76.1788, -0.2655)
  point P115 (75.2636, -0.2818)
  point P116 (74.3489, -0.299)
  point P117 (73.4349, -0.317)
  point P118 (72.5214, -0.3358)
  point P119 (71.6084, -0.3555)
  point P120 (70.6961, -0.3761)
  point P121 (69.7842, -0.3975)
  point P122 (68.8729, -0.4197)
  point P123 (67.9622, -0.4428)
  point P124 (67.0519, -0.4668)
  point P125 (66.1422, -0.4915)
  point P126 (65.233, -0.5171)
  point P127 (64.3243, -0.5435)
  point P128 (63.4161, -0.5707)
  point P129 (62.5084, -0.5987)
  point P130 (61.6012, -0.6274)
  point P131 (60.6944, -0.6569)
  point P132 (59.7881, -0.6871)
  point P133 (58.8822, -0.7181)
  point P134 (57.9769, -0.7497)
  point P135 (57.0719, -0.7819)
  point P136 (56.1674, -0.8148)
  point P137 (55.2633, -0.8483)
  point P138 (54.3596, -0.8823)
  point P139 (53.4564, -0.9169)
  point P140 (52.5535, -0.9519)
  point P141 (51.6511, -0.9874)
  point P142 (50.749, -1.0233)
  point P143 (49.8473, -1.0596)
  point P144 (48.946, -1.0962)
  point P145 (48.045, -1.1331)
  point P146 (47.1443, -1.1702)
  point P147 (46.244, -1.2074)
  point P148 (45.344, -1.2448)
  point P149 (44.4443, -1.2821)
  point P150 (43.545, -1.3195)
  point P151 (42.6459, -1.3568)
  point P152 (41.747, -1.3939)
  point P153 (40.8485, -1.4308)
  point P154 (39.9501, -1.4674)
  point P155 (39.052, -1.5037)
  point P156 (38.1542, -1.5394)
  point P157 (37.2565, -1.5746)
  point P158 (36.359, -1.6091)
  point P159 (35.4704, -1.6433)
  point P160 (34.5881, -1.6789)
  point P161 (33.706, -1.716)
  point P162 (32.8241, -1.7545)
  point P163 (31.9424, -1.7942)
  point P164 (31.0608, -1.835)
  point P165 (30.1792, -1.8768)
  point P166 (29.2977, -1.9194)
  point P167 (28.4161, -1.9627)
  point P168 (27.5343, -2.0066)
  point P169 (26.6523, -2.0508)
  point P170 (25.7701, -2.0952)
  point P171 (24.8875, -2.1396)
  point P172 (24.0045, -2.1838)
  point P173 (23.1209, -2.2275)
  point P174 (22.2367, -2.2706)
  point P175 (21.3518, -2.3128)
  point P176 (20.466, -2.3538)
  point P177 (19.5793, -2.3933)
  point P178 (18.6915, -2.4309)
  point P179 (17.8025, -2.4663)
  point P180 (16.9121, -2.4991)
  point P181 (16.0203, -2.5288)
  point P182 (15.1267, -2.5549)
  point P183 (14.2312, -2.5769)
  point P184 (13.3336, -2.5939)
  point P185 (12.4336, -2.6052)
  point P186 (11.531, -2.6099)
  point P187 (10.6253, -2.6069)
  point P188 (9.7163, -2.5947)
  point P189 (8.8034, -2.5716)
  point P190 (7.8861, -2.5354)
  point P191 (6.9635, -2.4832)
  point P192 (6.0348, -2.411)
  point P193 (5.0985, -2.3133)
  point P194 (4.1527, -2.1812)
  point P195 (3.194, -2.0002)
  point P196 (2.2163, -1.7418)
  point P197 (1.2039, -1.3327)
  dimension "d2" = 8
  dimension "d3" = 3.09
  dimension "d5" = 22.5
  dimension "d8" = 3.25
  dimension "d9" = 28
  constraint horizontal L0
  constraint vertical L1
  constraint coincident A0.centre L2.start
  constraint coincident A1.centre L2.end
  constraint parallel L0 L2
  measures "d2" diameter of A0
  measures "d3" distance of A0.centre L0
  measures "d5" distance of A0.centre L1
  measures "d8" diameter of A1
  measures "d9" distance of A0.centre A1.centre
extrude "Extrusion1" add sketch "Esquisse7" along normal blind 188
named bodies: "NACA4412"
